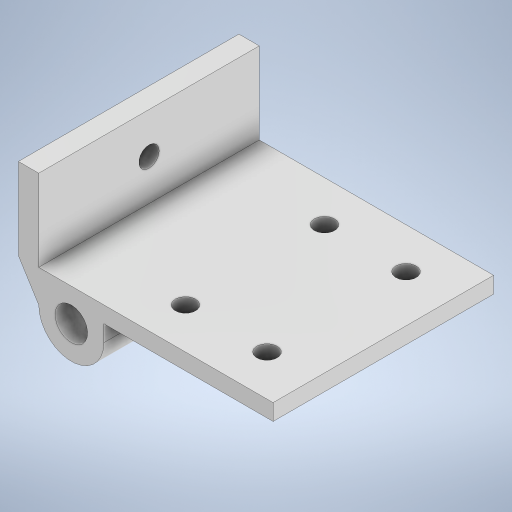
# Autodesk Inventor part: 4x2020_subaxis
Saved by Autodesk Inventor 2024 (Build 280153000, 153)
## iProperties
Created: 2025-12-25
Part Number: 4x2020_subaxis
Material: PET Plastic
Document SubType Name: Modeling
Designer: schar
Density: 1.541 g/cm^3
Appearance: Polycarbonate - Clear
Author: schar
Autodesk Inventor part; units mm, degrees
ref_plane "YZ Plane" through (0, 0, 0) normal (1, 0, 0) x (0, 1, 0)
ref_plane "XZ Plane" through (0, 0, 0) normal (0, 1, 0) x (-1, 0, 0)
ref_plane "XY Plane" through (0, 0, 0) normal (0, 0, 1) x (1, 0, 0)
sketch "Sketch1" plane through (0, 0, 0) normal (0, 1, 0) x (-1, 0, 0)
  line L0 (0, 0) -> (-50, 0)
  line L1 (-50, 0) -> (-50, -54.112)
  line L2 (-50, -54.112) -> (0, -54.112)
  line L3 (0, -54.112) -> (0, 0)
  dimension "d0" = 50
  dimension "d1" = 54.112
  constraints: 8 end point, 2 parallel, 1 horizontal, 1 perpendicular
  measures "d0" distance of L2.end L1.end
  measures "d1" distance of L1.end L0.end
extrude "Extrusion1" add sketch "Sketch1" along normal blind 4
sketch "Sketch2" plane through (50, 0, -54.112) normal (0, 0, -1) x (-1, 0, 0)
  line L0 (50, 0) -> (42, 0)
  line L1 (0, 0) -> (50, 0) projected
  line L2 (42, 0) -> (42, -4)
  circle A0 centre (42, -4) radius 4
  circle A1 centre (42, -4) radius 8
  line L3 (50, -4) -> (50, 0)
  line L4 (34, -4) -> (34, 0)
  line L5 (34, 0) -> (35.0718, 0)
  line L6 (50, 0) -> (48.9282, 0)
  dimension "d4" = 8
  dimension "d6" = 4
  dimension "d7" = 16
  constraints: 12 end point, 5 point on line, 4 point on circle, 2 coincident, 2 perpendicular, 2 tangent, 1 centre point, 1 vertical, 1 vertical alignment, 2 other
  measures "d4" distance of L0.start L0.end
  measures "d6" distance of L0.end L2.end
  measures "d7" diameter of A1
extrude "Extrusion2" add sketch "Sketch2" against normal blind 54.112 contours L3 A1 L0 | A1 L1 L0 | A1 L4 L1 picked at (48.5892, -4.6382)
sketch "Sketch4" plane through (0, 0, 0) normal (0, -1, 0) x (1, 0, 0)
  line L0 (50, -54.112) -> (16, -54.112) projected
  line L1 (16, -54.112) -> (26, -54.112)
  line L2 (26, -54.112) -> (26, -44.112)
  line L3 (0, 0) -> (50, 0) projected
  line L4 (26, 0) -> (16, 0)
  line L5 (26, 0) -> (26, -10)
  line L6 (26, -10) -> (46, -10)
  line L7 (26, -44.112) -> (46, -44.112)
  circle A0 centre (46, -44.112) radius 2.5
  circle A1 centre (46, -10) radius 2.5
  circle A2 centre (26, -10) radius 2.5
  circle A3 centre (26, -44.112) radius 2.5
  dimension "d10" = 10
  dimension "d11" = 10
  dimension "d12" = 10
  dimension "d13" = 10
  dimension "d14" = 20
  dimension "d15" = 20
  dimension "d16" = 5
  dimension "d17" = 5
  dimension "d18" = 5
  dimension "d19" = 5
  constraints: 12 end point, 4 centre point, 4 coincident, 3 point on line, 2 horizontal, 1 perpendicular, 1 vertical
  measures "d10" distance of L0.end L1.end
  measures "d11" distance of L1.end L2.end
  measures "d12" distance of L4.start L4.end
  measures "d13" distance of L4.start L5.end
  measures "d14" distance of L5.end L6.end
  measures "d15" distance of L2.end L7.end
  measures "d16" diameter of A0
  measures "d17" diameter of A1
  measures "d18" diameter of A2
  measures "d19" diameter of A3
extrude "Extrusion3" cut sketch "Sketch4" against normal blind 54.112
sketch "Sketch5" plane through (0, 4, -54.112) normal (-1, 0, 0) x (0, 0, 1)
  line L0 (0, 0) -> (54.112, 0) projected
  line L1 (0, 0) -> (54.112, 0)
  line L2 (54.112, 0) -> (54.112, 20)
  line L3 (54.112, 20) -> (0, 20)
  line L4 (0, 20) -> (0, 0)
  point P0 (54.112, -4)
  dimension "d22" = 20
  constraints: 8 end point, 2 parallel, 1 horizontal, 1 perpendicular
  measures "d22" distance of L2.end L1.end
extrude "Extrusion4" add sketch "Sketch5" along normal blind 5
sketch "Sketch6" plane through (50, 0, 0) normal (0, 0, 1) x (1, 0, 0)
  line L0 (-50, 4) -> (-55, 4) projected
  line L1 (-50, -4) -> (-50, 4) projected
  line L2 (-55, 4) -> (-50, -4)
  line L3 (-50, -4) -> (-50, 4)
  line L4 (-50, 4) -> (-55, 4)
  point P0 (-50, 0)
  constraints: 6 end point, 1 collinear, 1 perpendicular
extrude "Extrusion5" add sketch "Sketch6" against normal up to surface (54.112 mm away)
sketch "Sketch7" plane through (-5, 4, -54.112) normal (-1, 0, 0) x (0, 0, 1)
  line L0 (0, 0) -> (54.112, 0) projected
  line L1 (0, 0) -> (27.056, 0)
  line L2 (27.056, 0) -> (27.056, 10)
  circle A0 centre (27.056, 10) radius 2.5
  point P0 (54.112, -4)
  dimension "d27" = 10
  dimension "d28" = 5
  constraints: 4 end point, 1 centre point, 1 coincident, 1 midpoint, 1 perpendicular
  measures "d27" distance of L1.end L2.end
  measures "d28" diameter of A0
extrude "Extrusion6" cut sketch "Sketch7" against normal blind 10
sketch "Sketch8" plane through (50, 0, 0) normal (1, 0, 0) x (0, 0, -1)
  line L0 (54.112, 4) -> (0, 4) projected
  line L1 (0, 0) -> (54.112, 0) projected
  line L2 (0, 4) -> (54.112, 4)
  line L3 (54.112, 4) -> (54.112, 0)
  line L4 (54.112, 0) -> (0, 0)
  line L5 (0, 0) -> (0, 4)
  constraints: 8 end point, 2 parallel, 1 horizontal, 1 perpendicular
extrude "Extrusion7" add sketch "Sketch8" along normal blind 7.5
body "Solid1"
